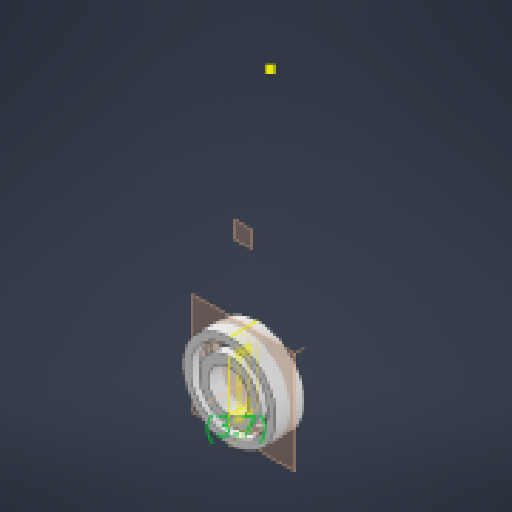
# Autodesk Inventor part: custom_bearing
Saved by Autodesk Inventor 2026.1 (Build 301233020, 233B)
## iProperties
Created: 2025-11-24
Part Number: custom_bearing
Material: 일반
Document SubType Name: Modeling
Designer: jaewook
Density: 1 g/cm^3
Appearance: 기본값
Author: jaewook
Autodesk Inventor part; units mm, degrees
ref_plane "YZ Plane" through (0, 0, 0) normal (1, 0, 0) x (0, 1, 0)
ref_plane "XZ Plane" through (0, 0, 0) normal (0, 1, 0) x (-1, 0, 0)
ref_plane "XY Plane" through (0, 0, 0) normal (0, 0, 1) x (1, 0, 0)
ref_plane "작업 평면1" through (0, -41, 8.5) normal (0, 0, 1) x (1, 0, 0)
sketch "스케치1" plane through (0, -41, 8.5) normal (0, 0, 1) x (1, 0, 0)
  circle A0 centre (0, -40.5) radius 15 projected
  circle A1 centre (0, -40.5) radius 5 projected
  circle A2 centre (0, -40.5) radius 14.7
  circle A3 centre (0, -40.5) radius 5.3
  circle A4 centre (0, -40.5) radius 13
  circle A5 centre (0, -40.5) radius 7
  point P0 (0, 41)
  dimension "d0" = 0.3
  dimension "d1" = 0.3
  dimension "d2" = 1.7
  dimension "d3" = 1.7
  constraints: 4 centre point
  measures "d0" radial gap between concentric circles of A0 A2
  measures "d1" radial gap between concentric circles of A1 A3
  measures "d2" radial gap between concentric circles of A3 A5
  measures "d3" radial gap between concentric circles of A2 A4
extrude "돌출1" add sketch "스케치1" along normal mid plane 9 contours A2 | A5
ref_plane "작업 평면2" through (0, -81.5, 8.5) normal (0, 0, 1) x (1, 0, 0)
sketch "스케치3" plane through (0, -81.5, 13) normal (0, 0, 1) x (1, 0, 0)
  circle A0 centre (0, 0) radius 13 projected
  circle A1 centre (0, 0) radius 12
  circle A2 centre (0, 0) radius 7 projected
  circle A3 centre (0, 0) radius 8
  point P0 (0, 81.5)
  dimension "d11" = 1
  dimension "d12" = 1
  constraints: 2 centre point
  measures "d11" radial gap between concentric circles of A0 A1
  measures "d12" radial gap between concentric circles of A2 A3
extrude "돌출2" add sketch "스케치3" against normal blind 2.3
mirror "미러1" about plane through (0, -81.5, 8.5) normal (0, 0, 1) of "돌출2"
sketch "스케치4" plane through (0, 0, 0) normal (1, 0, 0) x (0, 1, 0)
  line L0 (-76.2, 4) -> (-86.8, 4) projected
  line L1 (-86.8, 13) -> (-76.2, 13) projected
  line L2 (-74.5, 6.3) -> (-88.5, 6.3) construction
  line L3 (-88.5, 10.7) -> (-74.5, 10.7) projected
  line L4 (-86.8, 13) -> (-86.8, 4) projected
  line L5 (-76.2, 13) -> (-76.2, 4) projected
  line L6 (-94.5, 10.7) -> (-94.5, 6.3) projected
  line L7 (-66.8, 4) -> (-66.8, 13) projected
  line L8 (-96.2, 4) -> (-96.2, 13) projected
  line L9 (-68.5, 10.7) -> (-68.5, 6.3) projected
  line L10 (-73.5, 13) -> (-89.5, 13) projected
  line L11 (-73.5, 4) -> (-89.5, 4) projected
  line L12 (-89.5, 6.3) -> (-89.5, 4) projected
  line L13 (-89.5, 13) -> (-89.5, 10.7) projected
  line L14 (-68.5, 10.7) -> (-94.5, 10.7) projected
  line L15 (-94.5, 6.3) -> (-68.5, 6.3) projected
  line L16 (-94.5, 10.7) -> (-94.5, 6.3) projected
  line L17 (-89.5, 10.7) -> (-73.5, 10.7) projected
  line L18 (-89.5, 6.3) -> (-73.5, 6.3) projected
  point P0 (0, 0)
  point P1 (-90.4, 10)
  point P2 (-72.6, 10)
  point P3 (-90.4, 7)
  point P4 (-72.6, 7)
  point P5 (-72.6, 9.7)
  point P6 (-90.4, 9.7)
  point P7 (-90.4, 7.3)
  point P8 (-72.6, 7.3)
  point P9 (-89.8, 10)
  point P10 (-73.2, 10)
  point P11 (-89.8, 7)
  point P12 (-73.2, 7)
  dimension "d15" = 5
  constraints: 4 other
sketch "스케치5" plane through (0, -81.5, 4) normal (0, 0, -1) x (-1, 0, 0)
  circle A0 centre (0, 0) radius 12 projected
  circle A1 centre (0, 0) radius 11.8
  point P0 (0, 81.5)
  dimension "d16" = 0.2
  constraints: 1 centre point
  measures "d16" radial gap between concentric circles of A0 A1
extrude "돌출3" add sketch "스케치5" against normal blind 2.3
